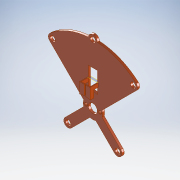
# Autodesk Inventor part: Pok Yaw Motor Face Mount
Saved by Autodesk Inventor 2018.2 (Build 222227000, 227)
## iProperties
Created: 2018-02-07
Part Number: Pok Yaw Motor Face Mount
Material: ABS Plastic
Document SubType Name: Modeling
Designer: Moochster
Density: 1.06 g/cm^3
Appearance: Smooth - Light Orange
Author: Moochster
Autodesk Inventor part; units mm, degrees
ref_plane "YZ Plane" through (0, 0, 0) normal (1, 0, 0) x (0, 1, 0)
ref_plane "XZ Plane" through (0, 0, 0) normal (0, 1, 0) x (-1, 0, 0)
ref_plane "XY Plane" through (0, 0, 0) normal (0, 0, 1) x (1, 0, 0)
sketch "Sketch1" plane through (0, 0, 0) normal (0, 1, 0) x (-1, 0, 0)
  circle A0 centre (0, 0) radius 5 construction
  circle A1 centre (0, 0) radius 5.15
  circle A2 centre (8, 0) radius 1.25
  circle A3 centre (-8, 0) radius 1.25
  circle A4 centre (0, 0) radius 15 construction
  arc A5 (15.0247, 7.9536) -> (5.15, 16.2012) centre (0, 0) ccw
  arc A6 (5.7403, 13.8582) -> (-5.7403, 13.8582) centre (0, 0) ccw construction
  line L0 (6.5056, 15.706) -> (5.7403, 13.8582) construction
  line L1 (-5.7403, 13.8582) -> (-6.5056, 15.706) construction
  line L2 (3, 14.6969) -> (3, 10.583) construction
  line L3 (-3, 14.6969) -> (-3, 10.583) construction
  line L4 (5, 16.2481) -> (5, 28) construction
  line L5 (5, 28) -> (-5, 28) construction
  line L6 (-5, 28) -> (-5, 16.2481) construction
  line L7 (5.15, 16.2012) -> (5.15, 40.2012)
  line L8 (5.15, 40.2012) -> (-5.15, 40.2012)
  line L9 (-5.15, 40.2012) -> (-5.15, 16.2012)
  line L10 (0, 0) -> (28.2843, -28.2843) construction
  line L11 (0, 0) -> (33.0235, 0) construction
  circle A7 centre (28.2843, -28.2843) radius 3
  line L12 (3.3927, -10.4637) -> (6.4645, -13.5355)
  arc A8 (24.7487, -31.8198) -> (31.8198, -24.7487) centre (28.2843, -28.2843) ccw
  line L13 (31.8198, -24.7487) -> (15.0247, -7.9536)
  line L14 (0, 0) -> (0, -40.6954) construction
  circle A9 centre (-28.2843, -28.2843) radius 3
  line L15 (-3.3927, -10.4637) -> (-24.7487, -31.8198)
  arc A10 (-31.8198, -24.7487) -> (-24.7487, -31.8198) centre (-28.2843, -28.2843) ccw
  line L16 (-31.8198, -24.7487) -> (-10.4637, -3.3927)
  line L17 (0, 0) -> (-45.9619, 45.9619) construction
  circle A11 centre (-45.9619, 45.9619) radius 3
  line L18 (-10.4637, 3.3927) -> (-15.0247, 7.9536)
  line L19 (0, 0) -> (0, 70) construction
  arc A12 (-49.4975, 49.4975) -> (-49.4975, 42.4264) centre (-45.9619, 45.9619) ccw
  circle A13 centre (45.9619, 45.9619) radius 3
  line L20 (10.4637, 3.3927) -> (15.0247, 7.9536)
  arc A14 (49.4975, 42.4264) -> (49.4975, 49.4975) centre (45.9619, 45.9619) ccw
  line L21 (7.9536, -15.0247) -> (24.7487, -31.8198)
  line L22 (6.4645, -13.5355) -> (7.9536, -15.0247)
  line L23 (15.0247, -7.9536) -> (13.5355, -6.4645)
  line L24 (13.5355, -6.4645) -> (10.4637, -3.3927)
  arc A15 (-3.3927, -10.4637) -> (3.3927, -10.4637) centre (0, 0) ccw
  circle A16 centre (0, 70) radius 3
  circle A17 centre (0, 70) radius 5
  arc A18 (-5.15, 16.2012) -> (-15.0247, 7.9536) centre (0, 0) ccw
  arc A19 (5.15, 16.2012) -> (5, 16.2481) centre (0, 0) ccw
  arc A20 (-10.4637, -3.3927) -> (-3.3927, -10.4637) centre (0, 0) ccw
  arc A21 (3.3927, -10.4637) -> (10.4637, -3.3927) centre (0, 0) ccw
  arc A22 (10.4637, -3.3927) -> (10.4637, 3.3927) centre (0, 0) ccw
  arc A23 (-5, 16.2481) -> (-5.15, 16.2012) centre (0, 0) ccw
  arc A24 (5, 16.2481) -> (-5, 16.2481) centre (0, 0) ccw
  line L25 (15.0247, 7.9536) -> (49.4975, 42.4264)
  line L26 (-15.0247, 7.9536) -> (-49.4975, 42.4264)
  arc A25 (-10.4637, 3.3927) -> (-10.4637, -3.3927) centre (0, 0) ccw
  arc A26 (10.4637, 3.3927) -> (-10.4637, 3.3927) centre (0, 0) ccw
  arc A27 (49.4975, 49.4975) -> (4.9968, 69.8214) centre (0, 0) ccw
  arc A28 (-4.9968, 69.8214) -> (-49.4975, 49.4975) centre (0, 0) ccw
  arc A29 (-2.9993, 69.9357) -> (-4.9968, 69.8214) centre (0, 0) ccw construction
  arc A30 (2.9993, 69.9357) -> (-2.9993, 69.9357) centre (0, 0) ccw construction
  arc A31 (4.9968, 69.8214) -> (2.9993, 69.9357) centre (0, 0) ccw construction
  point P0 (0, 17)
  point P1 (0, 28)
  dimension "d0" = 10
  dimension "d1" = 0.15
  dimension "d2" = 2.5
  dimension "d4" = 8
  dimension "d5" = 8
  dimension "d14" = 2
  dimension "d15" = 6
  dimension "d16" = 45
  dimension "d47" = 10
  dimension "d48" = 11
  dimension "d56" = 0.15
  dimension "d57" = 0.15
  dimension "d58" = 24
  dimension "d61" = 45
  dimension "d62" = 40
  dimension "d63" = 5
  dimension "d64" = 6
  dimension "d69" = 45
  dimension "d70" = 65
  dimension "d71" = 6
  dimension "d72" = 5
  dimension "d104" = 22
  dimension "d105" = 4
  dimension "d106" = 6
  dimension "d108" = 17
  dimension "d132" = 10
  constraints: 78 point on circle, 54 end point, 31 centre point, 13 parallel, 11 symmetric about line, 10 tangent, 7 coincident, 7 vertical, 5 concentric, 3 horizontal alignment, 3 perpendicular, 3 point on line, 2 vertical alignment, 1 equal radius, 1 horizontal, 1 midpoint, 9 other
  measures "d0" diameter of A0
  measures "d1" radial gap between concentric circles of A0 A1
  measures "d2" diameter of A2
  measures "d4" distance of L10.start A2.centre
  measures "d5" distance of A3.centre L10.start
  measures "d14" radial gap between concentric circles of A5 A6
  measures "d15" distance between parallel lines of L2 L3
  measures "d16" angle of L0 L1
  measures "d47" distance of L4.end L5.end
  measures "d48" distance from line of point (0, 17) L5
  measures "d56" distance between parallel lines of L6 L9
  measures "d57" distance between parallel lines of L7 L4
  measures "d58" distance of L7.start L7.end
  measures "d61" angle of L10 L11
  measures "d62" distance of L10.start L10.end
  measures "d63" radius of A8
  measures "d64" diameter of A7
  measures "d69" angle of L17 L14
  measures "d70" distance of L17.start L17.end
  measures "d71" diameter of A11
  measures "d72" radius of A12
  measures "d104" diameter of A15
  measures "d106" diameter of A16
  measures "d108" radius of A5
  measures "d132" diameter of A17
extrude "Extrusion11" add sketch "Sketch1" along normal blind 2.5 contours L20 A26 L18 A18 A23 A24 A19 A5 | A5 L7 L8 L9 A18 L26 A12 A28 A17 A27 A14 L25 | A22 A21 A15 A20 A25 A26 | L24 L23 L13 A8 L21 L22 L12 A21 | A20 L15 A10 L16 | A17
chamfer "Chamfer1" distance 0.5 angle 45 2 edges at (9.25, 0, 0) (-6.75, 0, 0)
ref_plane "Work Plane5" through (5.15, 0, 28.2012) normal (0, 0, -1) x (-1, 0, 0)
sketch "Sketch9" plane through (5.15, 0, 28.2012) normal (0, 0, -1) x (-1, 0, 0)
  line L0 (-4.6, 0) -> (-1.1, 0) projected
  line L1 (-20.1343, 0) -> (-26.1343, 0) projected
  line L2 (10.3, 0) -> (0, 0) projected
  line L3 (36.4343, 0) -> (30.4343, 0) projected
  line L4 (-44.3475, 0) -> (-5.3137, 0) projected
  line L5 (15.6137, 0) -> (54.6475, 0) projected
  line L6 (15.6137, 0) -> (15.6137, 0) projected
  line L7 (36.9698, 0) -> (15.6137, 0) projected
  line L8 (29.8987, 0) -> (36.9698, 0) projected
  line L9 (8.5427, 0) -> (29.8987, 0) projected
  line L10 (1.7573, 0) -> (8.5427, 0) projected
  line L11 (-19.5987, 0) -> (1.7573, 0) projected
  line L12 (-26.6698, 0) -> (-19.5987, 0) projected
  line L13 (-5.3137, 0) -> (-26.6698, 0) projected
  line L14 (-5.3137, 0) -> (-5.3137, 0) projected
  line L15 (11.4, 0) -> (14.9, 0) projected
  line L16 (-19.5987, 0) -> (1.7573, 0) projected
  line L17 (0.15, 0) -> (0.15, -8.2)
  line L18 (0.15, -8.2) -> (4.4, -8.2)
  line L19 (4.4, -8.2) -> (4.4, -9.2)
  line L20 (4.4, -9.2) -> (-0.85, -9.2)
  line L21 (-0.85, -9.2) -> (-0.85, 0)
  line L22 (11.4, 0) -> (14.9, 0) projected
  line L23 (11.15, 0) -> (11.15, -9.2)
  line L24 (11.15, -9.2) -> (5.9, -9.2)
  line L25 (5.9, -9.2) -> (5.9, -8.2)
  line L26 (5.9, -8.2) -> (10.15, -8.2)
  line L27 (10.15, -8.2) -> (10.15, 0)
  line L28 (11.15, 0) -> (10.15, 0)
  line L29 (0.15, 0) -> (-0.85, 0)
  line L30 (13.8526, 4) -> (-4.1953, 4) construction
  line L31 (0.1532, 0) -> (10.1468, 0) projected
  line L32 (54.6475, 0) -> (10.1468, 0) projected
  line L33 (54.6475, 0) -> (54.6475, 0) projected
  line L34 (-44.3475, 0) -> (-44.3475, 0) projected
  line L35 (0.1532, 0) -> (-44.3475, 0) projected
  line L36 (10.3, 2.5) -> (0, 2.5) projected
  point P0 (5.15, 0)
  point P1 (0.1528, 0)
  point P2 (-37.8119, 0)
  point P3 (-43.8119, 0)
  point P4 (54.1119, 0)
  point P5 (48.1119, 0)
  point P6 (2.15, 0)
  point P7 (8.15, 0)
  dimension "d117" = 1.5
  dimension "d118" = 10
  dimension "d119" = 5
  dimension "d121" = 1
  dimension "d122" = 1
  dimension "d125" = 12.2
  dimension "d133" = 1.5
  constraints: 26 end point, 8 perpendicular, 6 point on line, 3 collinear, 1 horizontal, 1 parallel, 3 other
  measures "d117" distance between parallel lines of L19 L25
  measures "d118" distance between parallel lines of L17 L27
  measures "d119" distance from line of point (5.15, 0) L27
  measures "d121" distance of L18.end L19.end
  measures "d122" distance between parallel lines of L17 L21
  measures "d125" distance between parallel lines of L26 L30
  measures "d133" distance between parallel lines of L36 L30
extrude "Extrusion12" add sketch "Sketch9" along normal up to surface round surface about axis through (0, 0, 0) along (0, 1, 0) radius 17 far side no
sketch "Sketch10" plane through (-6, -9.2, 28.2012) normal (-1, 0, 0) x (0, 0, 1)
  line L0 (-12.2952, 9.2) -> (-12, 9.2) projected
  line L1 (-12.2952, 9.2) -> (-4.2952, 9.2)
  line L2 (-4.2952, 9.2) -> (-4.2952, 4.2)
  line L3 (-4.2952, 4.2) -> (-12.2952, 4.2)
  line L4 (-12.2952, 4.2) -> (-12.2952, 9.2)
  point P0 (-28.2012, 9.2)
  dimension "d128" = 8
  dimension "d129" = 5
  constraints: 8 end point, 2 parallel, 1 horizontal, 1 perpendicular
  measures "d128" distance of L2.end L3.end
  measures "d129" distance of L1.end L2.end
extrude "Extrusion13" cut sketch "Sketch10" against normal through all
body "Solid2"
